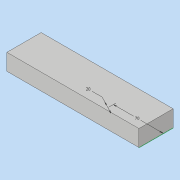
# Autodesk Inventor part: lw_6_part2
Saved by Autodesk Inventor 2019 (Build 230136000, 136)
## iProperties
Created: 2021-05-14
Part Number: lw_6_part2
Material: Типовые
Document SubType Name: Modeling
Designer: Kurbatova
Density: 1 g/cm^3
Appearance: По умолчанию
Author: Kurbatova
Autodesk Inventor part; units mm, degrees
ref_plane "YZ Plane" through (0, 0, 0) normal (1, 0, 0) x (0, 1, 0)
ref_plane "XZ Plane" through (0, 0, 0) normal (0, 1, 0) x (-1, 0, 0)
ref_plane "XY Plane" through (0, 0, 0) normal (0, 0, 1) x (1, 0, 0)
sketch "Эскиз1" plane through (0, 0, 0) normal (0, 0, 1) x (1, 0, 0)
  line L0 (-90.9717, -10.4774) -> (94.0283, -10.4774)
  line L1 (94.0283, -10.4774) -> (94.0283, 12.5226)
  line L2 (94.0283, 12.5226) -> (-90.9717, 12.5226)
  line L3 (-90.9717, 12.5226) -> (-90.9717, -10.4774)
  dimension "d2" = 185
  dimension "parametr_D" = 23
  constraints: 8 end point, 2 perpendicular, 1 horizontal, 1 vertical
  measures "d2" distance of L0.start L0.end
  measures "parametr_D" distance of L0.end L1.end
extrude "Выдавливание1" add sketch "Эскиз1" along normal blind 48
sketch "Эскиз2" plane through (-90.9717, -10.4774, 0) normal (0, -1, 0) x (1, 0, 0)
  circle A0 centre (115, 21.3555) radius 10
  line L0 (185, 0) -> (185, 48) projected
  point P0 (90.9717, 0)
  dimension "d9" = 20
  dimension "d11" = 70
  constraints: 1 centre point
  measures "d9" diameter of A0
  measures "d11" distance from line of L0 A0.centre
equation "\"d2\" = parametr_A_"
equation "\"d4\" = parametr_B_"
equation "\"parametr_A_\" = 185"
equation "\"parametr_B_\" = 48"
